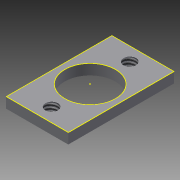
# Autodesk Inventor part: recessedCoverslipHolder_v1
Saved by Autodesk Inventor 2013 (Build 170138000, 138)
## iProperties
Created: 2014-12-18
Part Number: recessedCoverslipHolder_v1
Material: Generic
Document SubType Name: Modeling
Designer: 120pa
Density: 1 g/cm^3
Author: 120pa
Autodesk Inventor part; units mm, degrees
ref_plane "YZ Plane" through (0, 0, 0) normal (1, 0, 0) x (0, 1, 0)
ref_plane "XZ Plane" through (0, 0, 0) normal (0, 1, 0) x (-1, 0, 0)
ref_plane "XY Plane" through (0, 0, 0) normal (0, 0, 1) x (1, 0, 0)
sketch "Sketch2" plane through (0, 0, 0) normal (0, 1, 0) x (-1, 0, 0)
  line L0 (0, 0) -> (5.881, 0)
  line L1 (5.881, 0) -> (5.881, 10)
  line L2 (5.881, 10) -> (0, 10)
  line L3 (0, 10) -> (0, 0)
  dimension "d2" = 5.881
  dimension "d3" = 10
  constraints: 8 end point
  measures "d2" distance of L2.end L1.end
  measures "d3" distance of L1.end L0.end
extrude "Extrusion2" add sketch "Sketch2" along normal blind 1
sketch "Sketch3" plane through (0, 1, 0) normal (0, 1, 0) x (1, 0, 0)
  circle A0 centre (-2.9405, -5) radius 2.4
  dimension "d6" = 4.8
  constraints: 1 centre point
  measures "d6" diameter of A0
extrude "Extrusion3" cut sketch "Sketch3" against normal blind 1
sketch "Sketch4" plane through (0, 1, 0) normal (0, 1, 0) x (1, 0, 0)
  circle A0 centre (-2.9405, -5) radius 2.4 projected
  line L0 (0, 0) -> (-5.881, 0) projected
  line L1 (-5.881, 0) -> (-5.881, -10) projected
  line L2 (-5.881, -10) -> (0, -10) projected
  line L3 (0, -10) -> (0, 0) projected
hole "Hole1" at (-2.881, 1, 1.3) direction (0, -1, 0) diameter 1.181 end through all thread size "0-80 UNF" class "2B" standard "ANSI Unified Screw Threads"
hole "Hole2" at (-2.881, 1, 8.7) direction (0, -1, 0) diameter 1.181 end through all thread size "0-80 UNF" class "2B" standard "ANSI Unified Screw Threads"
body "Solid2"
